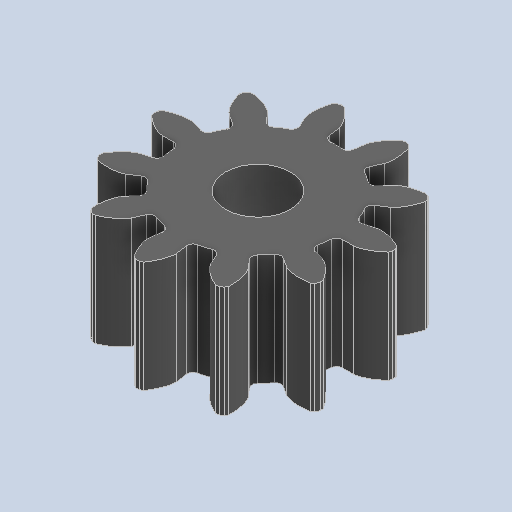
# Autodesk Inventor part: screw_middle_gear_under_12
Saved by Autodesk Inventor 2024.1 (Build 281209000, 209)
## iProperties
Created: 2025-01-10
Part Number: screw_middle_gear_under_12
Material: 一般
Document SubType Name: Modeling
Designer: hibik
Density: 1 g/cm^3
Appearance: 既定
Author: hibik
Autodesk Inventor part; units mm, degrees
ref_plane "YZ Plane" through (0, 0, 0) normal (1, 0, 0) x (0, 1, 0)
ref_plane "XZ Plane" through (0, 0, 0) normal (0, 1, 0) x (-1, 0, 0)
ref_plane "XY Plane" through (0, 0, 0) normal (0, 0, 1) x (1, 0, 0)
sketch "スケッチ1" plane through (0, 0, 0) normal (0, 1, 0) x (-1, 0, 0)
  circle A0 centre (0, 0) radius 5.5 construction
  circle A1 centre (0, 0) radius 5.1683 construction
  line L0 (0, 0) -> (0.7355, -5.1157)
  line L1 (0, -9.5924) -> (0, 8.0154) projected
  dimension "d1" = 10.3366
  dimension "d0" = 11
  dimension "d4" = 8.182
  constraints: 3 coincident, 2 end point, 1 centre point, 7 other
  measures "d0" diameter of A0
  measures "d4" angle of L1 L0
sketch "スケッチ2" plane through (0, 0, 0) normal (0, 1, 0) x (-1, 0, 0)
  circle A0 centre (0, 0) radius 6.5
  dimension "d5" = 13
  constraints: 1 centre point, 1 coincident
  measures "d5" diameter of A0
extrude "押し出し1" add sketch "スケッチ2" along normal blind 6
sketch "スケッチ3" plane through (0, 6, 0) normal (0, 1, 0) x (1, 0, 0)
  line L0 (0, 0) -> (-0.7355, 5.1157) projected
  spline S0 degree 3 poles (-0.7355, 5.1157) (-0.7355, 5.1158) (-0.8126, 5.5427) (-1.3851, 6.0793) (-1.6608, 6.3379) (-2.0474, 6.6147) (-2.557, 6.8472) knots 0 0 0 0 0.674859 0.674859 0.674859 1 1 1 1 projected
  circle A0 centre (0, 0) radius 6.5 projected
  circle A1 centre (0, 0) radius 4.25
  line L1 (0, 9.7924) -> (0, -9.2154) projected
  point P0 (0, 4.25)
  point P1 (0, 6.5)
  point P2 (-1.6329, 6.2915)
  point P3 (-0.6048, 4.2067)
  dimension "d10" = 8.5
  constraints: 3 coincident, 1 centre point
  measures "d10" diameter of A1
extrude "押し出し2" cut sketch "スケッチ3" against normal through all contours L0 S0 A0 L1 A1 picked at (-0.2452, 5.2886)
fillet "フィレット1" radius 0.3 1 edges at (-0.6048, 3, -4.2067)
chamfer "面取り1" distance 0.1 angle 45 1 edges at (-1.6329, 3, -6.2915)
mirror "ミラー1" about plane through (0, 6, -6.5) normal (-1, 0, 0) of "押し出し2", "フィレット1", "面取り1"
pattern_circular "円形状パターン1" count 11 over 360 about axis through (0, -10, 0) along (0, 1, 0) of "押し出し2", "フィレット1", "面取り1", "ミラー1"
sketch "スケッチ6" plane through (0, 0, 0) normal (0, -1, 0) x (1, 0, 0)
  circle A0 centre (0, 0) radius 3.05
  dimension "d26" = 6.1
  constraints: 1 centre point, 1 coincident
  measures "d26" diameter of A0
extrude "押し出し5" cut sketch "スケッチ6" against normal blind 2.5
sketch "スケッチ10" plane through (0, 2.5, 0) normal (0, -1, 0) x (1, 0, 0)
  circle A0 centre (0, 0) radius 1.75
  dimension "d40" = 3.5
  constraints: 1 centre point, 1 coincident
  measures "d40" diameter of A0
extrude "押し出し9" cut sketch "スケッチ10" against normal through all
equation "\"module\" = 1"
